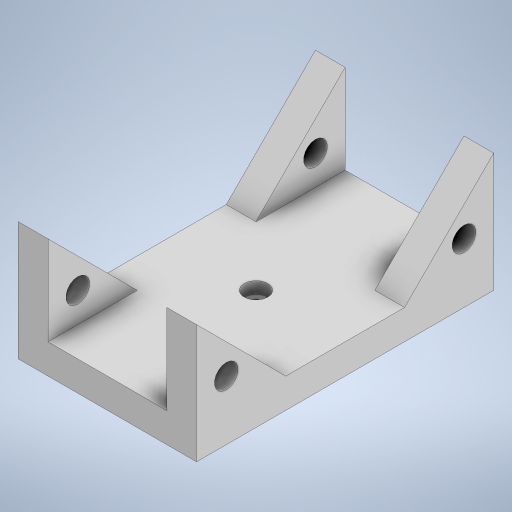
# Autodesk Inventor part: lower fan mount
Saved by Autodesk Inventor 2024 (Build 280153000, 153)
## iProperties
Created: 2023-05-15
Part Number: lower fan mount
Material: Generic
Document SubType Name: Modeling
Designer: skyfi
Density: 1 g/cm^3
Appearance: Default
Author: skyfi
Autodesk Inventor part; units mm, degrees
ref_plane "YZ Plane" through (0, 0, 0) normal (1, 0, 0) x (0, 1, 0)
ref_plane "XZ Plane" through (0, 0, 0) normal (0, 1, 0) x (-1, 0, 0)
ref_plane "XY Plane" through (0, 0, 0) normal (0, 0, 1) x (1, 0, 0)
sketch "Sketch1" plane through (0, 0, 0) normal (1, 0, 0) x (0, 1, 0)
  line L0 (15, 25) -> (-5, 25)
  line L1 (-5, 25) -> (-5, -25)
  line L2 (-5, -25) -> (15, -25)
  line L3 (15, -25) -> (0, -10)
  line L4 (0, -10) -> (0, 10)
  line L5 (0, 10) -> (15, 25)
  line L6 (0, 0) -> (-5, 0) construction
  circle A0 centre (5, -20) radius 2
  circle A1 centre (5, 20) radius 2
  dimension "d0" = 50
  dimension "d1" = 45
  dimension "d2" = 5
  dimension "d4" = 40
  dimension "d5" = 4
  dimension "d6" = 20
  dimension "d7" = 5
  dimension "d8" = 15
  constraints: 14 end point, 2 centre point, 2 equal length, 2 midpoint, 2 perpendicular, 1 coincident, 1 equal radius, 1 horizontal, 1 parallel, 1 vertical alignment
  measures "d0" distance of L0.end L1.end
  measures "d1" angle of L5 L0
  measures "d2" distance between parallel lines of L4 L1
  measures "d4" distance of A0.centre A1.centre
  measures "d5" diameter of A1
  measures "d6" vertical distance of point (0, 0) A0.centre
  measures "d7" distance from line of L4 A0.centre
  measures "d8" distance from line of L4 L2.end
extrude "Extrusion1" add sketch "Sketch1" along normal blind 5
sketch "Sketch2" plane through (0, 0, 0) normal (-1, 0, 0) x (0, 0, 1)
  line L0 (25, -5) -> (-25, -5) projected
  line L1 (-25, -5) -> (25, -5)
  line L2 (25, -5) -> (25, 0)
  line L3 (25, 0) -> (-25, 0)
  line L4 (-25, 0) -> (-25, -5)
  point P0 (0, 0)
  constraints: 8 end point, 2 parallel, 1 horizontal, 1 midpoint, 1 perpendicular
extrude "Extrusion2" add sketch "Sketch2" along normal blind 10
mirror "Mirror1" about plane through (-10, -2.5, 0) normal (-1, 0, 0)
sketch "Sketch3" plane through (0, 0, 10) normal (0, 1, 0) x (1, 0, 0)
  line L0 (-20, 0) -> (-20, -15) construction
  line L1 (0, 20) -> (5, 20) construction
  line L2 (-20, 0) -> (0, 20) construction
  line L3 (-20, 35) -> (-20, 20) construction
  line L4 (0, 0) -> (5, 0) construction
  line L5 (-20, 20) -> (0, 0) construction
  circle A0 centre (-10, 10) radius 2
  point P0 (0, 10)
  dimension "d13" = 4
  constraints: 4 end point, 1 centre point, 1 midpoint
  measures "d13" diameter of A0
extrude "Extrusion3" cut sketch "Sketch3" against normal blind 2
sketch "Sketch4" plane through (0, 0, 10) normal (0, 1, 0) x (1, 0, 0)
  circle A0 centre (-10, 10) radius 2 projected
  circle A1 centre (-10, 10) radius 1
  point P0 (0, 10)
  dimension "d16" = 2
  constraints: 1 centre point, 1 coincident
  measures "d16" diameter of A1
extrude "Extrusion4" cut sketch "Sketch4" against normal through all contours A1
equation "\"d6\" = 0.5 * d4"
equation "\"d7\" = 0.333333 * d8"
body "Solid1"
